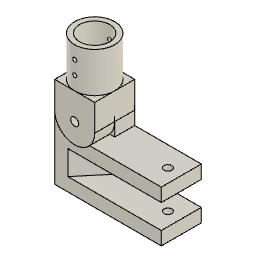
platform-bracket (Autodesk Fusion 360 design; units mm, degrees)
Autodesk Fusion 360 part; units mm, degrees
note: some values were not read from the file. Set by a fixed rule: which face or edge a step refers to.
sketch "Skizze2" plane through (0, 0, 0) normal (0, 0, 1) x (1, 0, 0)
  circle A0 centre (0, 0) radius 11.25
  circle A1 centre (0, 0) radius 15
  dimension "d1" = 22.5
  dimension "d2" = 30
  constraint coincident A0.centre A1.centre
  measures "d1" diameter of A0
  measures "d2" diameter of A1
extrude "Extrusion1" add sketch "Skizze2" along normal blind 30 makes body 1
sketch "Skizze3" plane through (0, 0, 0) normal (0, 0, -1) x (1, 0, 0)
  circle A0 centre (0, 0) radius 11.25
  circle A1 centre (0, 0) radius 15
  line L0 (15, -15) -> (-15, -15)
  line L1 (-15, -15) -> (-15, 15)
  line L2 (-15, 15) -> (15, 15)
  line L3 (15, 15) -> (15, -15)
  line L4 (15, -15) -> (-15, 15) construction
  line L5 (-15, -15) -> (15, 15) construction
  dimension "d5" = 30
  dimension "d6" = 30
  constraint perpendicular L0 L1
  constraint parallel L0 L2
  constraint parallel L1 L3
  constraint horizontal L0
  constraint coincident L4 A0.centre
  constraint coincident L5 A0.centre
  constraint coincident A0.centre A1.centre
  measures "d5" distance of L1.end L2.end
  measures "d6" distance of L0.end L1.end
extrude "Extrusion2" add sketch "Skizze3" along normal blind 5 contours A0 | A1 | A1 L0 L3 | A1 L2 L3 | A1 L1 L2 | A1 L0 L1 bodies 1
sketch "Skizze4" plane through (0, -15, 0) normal (0, -1, 0) x (1, 0, 0)
  line L0 (0, 0) -> (-15, 0)
  line L1 (-15, 0) -> (-15, -5)
  line L2 (-15, -5) -> (15, -5)
  line L3 (15, -5) -> (15, 0)
  line L4 (15, 0) -> (0, 0)
  circle A0 centre (0, -20) radius 15
  line L5 (-15, -5) -> (-15, -20)
  line L6 (15, -5) -> (15, -20)
  circle A1 centre (0, -20) radius 3
  dimension "d9" = 30
  dimension "d10" = 6
  constraint coincident L1.end L2.start
  constraint coincident A0 L5.end
  constraint tangent A0 L5
  constraint perpendicular L2 L5
  constraint coincident L2.end L3.start
  constraint coincident A0 L6.end
  constraint tangent A0 L6
  constraint perpendicular L2 L6
  constraint concentric A0 A1
  measures "d9" diameter of A0
  measures "d10" diameter of A1
extrude "Extrusion3" add sketch "Skizze4" against normal blind 15 contours L2 A0 L5 | L2 A0 L6 | A0 bodies 1
extrude "Extrusion4" add sketch "Skizze4" against normal blind 30 contours L2 A0 L5 | L2 A0 L6 bodies 1
sketch "Skizze5" plane through (0, 0, 0) normal (0, 1, 0) x (-1, 0, 0)
  arc A0 (15, -20) -> (-15, -20) centre (0, -20) ccw
  arc A1 (-15, -20) -> (15, -20) centre (0, -20) ccw
  circle A2 centre (0, -20) radius 3
  circle A3 centre (0, -20) radius 3
  circle A4 centre (0, -20) radius 15
  line L0 (15, -35) -> (-15, -35)
  line L1 (-15, -35) -> (-15, -5)
  line L2 (-15, -5) -> (15, -5)
  line L3 (15, -5) -> (15, -35)
  line L4 (15, -35) -> (-15, -5) construction
  line L5 (-15, -35) -> (15, -5) construction
  point P0 (0, -20)
  dimension "d15" = 30
  dimension "d16" = 30
  constraint concentric A0 A3
  constraint concentric A0 A4
  constraint coincident A0.start A4
  constraint perpendicular L0 L1
  constraint parallel L0 L2
  constraint parallel L1 L3
  constraint horizontal L0
  constraint coincident L4 P0
  constraint coincident L5 P0
  constraint coincident P0 A0.centre
  measures "d15" distance of L0.end L1.end
  measures "d16" distance of L1.end L2.end
extrude "Extrusion5" add sketch "Skizze5" along normal blind 15 separate body contours A0 A1 A4 | A1 A4 L0 L3 | A1 A4 L0 L1 makes body 2
extrude "Extrusion6" add sketch "Skizze5" against normal blind 15 contours A1 A4 L0 L3 | A1 A4 L0 L1 bodies 2
extrude "Extrusion7" add 3 faces at (0, 10, -35) (5, -5, -35) (-10, -10, -35) along direction (0, 0, -1) blind 5 on bodies 2 bodies 2
sketch "Skizze13" plane through (0, -15, 0) normal (0, -1, 0) x (1, 0, 0)
  line L0 (15, -40) -> (15, -20)
  arc A0 (-15, -20) -> (15, -20) centre (0, -20) ccw
  line L1 (-15, -20) -> (-15, -40)
  line L2 (-15, -40) -> (15, -40)
  line L3 (15, -30) -> (11.1803, -30)
  constraint midpoint L0 L3.start
  constraint coincident A0 L3.end
  constraint perpendicular L0 L3
extrude "Extrusion14" cut sketch "Skizze13" against normal blind 15 contours L0 A0 L3 bodies 2
sketch "Skizze14" plane through (15, 0, 0) normal (1, 0, 0) x (0, 1, 0)
  line L0 (0, -20) -> (0, -30)
  line L1 (0, -30) -> (-15, -30)
  line L2 (-15, -30) -> (-15, -40)
  line L3 (-15, -40) -> (15, -40)
  line L4 (15, -40) -> (15, -20)
  line L5 (15, -20) -> (0, -20)
  line L6 (0, -30) -> (15, -30)
  constraint coincident L0.end L1.start
  constraint midpoint L4 L6.end
extrude "Extrusion15" add sketch "Skizze14" along normal blind 50 contours L1 L2 L3 L4 L6 bodies 2
sketch "Skizze15" plane through (0, 0, -40) normal (0, 0, -1) x (1, 0, 0)
  line L0 (-15, 15) -> (-15, -15)
  line L1 (-15, -15) -> (65, -15)
  line L2 (65, -15) -> (65, 15)
  line L3 (65, 15) -> (-15, 15)
  line L4 (-15, 15) -> (-5, 15) construction
  circle A0 centre (577.121, 487.9008) radius 750
  dimension "d53" = 10
  dimension "d54" = 1500
  constraint coincident L0.start L3.end
  constraint perpendicular L0 L4
  constraint coincident L4.end A0
  measures "d53" distance of L0.start L4.end
  measures "d54" diameter of A0
extrude "Extrusion16" add sketch "Skizze15" along normal blind 18.2 contours L0 L1 L3 A0 bodies 2
sketch "Skizze16" plane through (0, 0, -58.2) normal (0, 0, -1) x (1, 0, 0)
  line L0 (-5, 15) -> (-15, 15)
  line L1 (-15, 15) -> (-15, -15)
  line L2 (-15, -15) -> (20.7121, -15)
  arc A0 (-5, 15) -> (20.7121, -15) centre (577.121, 487.9008) ccw
  line L3 (-15, 15) -> (65, 15)
  line L4 (65, 15) -> (65, -15)
  line L5 (65, -15) -> (-15, -15)
  line L6 (-15, -15) -> (-15, 15)
  dimension "d57" = 80
  dimension "d58" = 30
  constraint horizontal L3
  constraint vertical L4
  constraint horizontal L5
  constraint vertical L6
  constraint coincident L0.end L1.start
  measures "d57" distance of L0.end L3.end
  measures "d58" distance of L0.end L1.end
extrude "Extrusion17" add sketch "Skizze16" along normal blind 10 bodies 2
sketch "Skizze17" plane through (0, 0, -68.2) normal (0, 0, -1) x (1, 0, 0)
  line L0 (-15, -15) -> (65, -15)
  line L1 (65, -15) -> (65, 15)
  line L2 (65, 15) -> (-15, 15)
  line L3 (-15, 15) -> (-15, -15)
  line L4 (65, 0) -> (55, 0) construction
  circle A0 centre (55, 0) radius 3
  dimension "d61" = 10
  dimension "d62" = 6
  constraint midpoint L1 L4.start
  constraint perpendicular L1 L4
  constraint coincident L4.end A0.centre
  measures "d61" distance of L4.start L4.end
  measures "d62" diameter of A0
extrude "Extrusion18" cut sketch "Skizze17" against normal blind 40 contours A0 bodies 2
sketch "Skizze18" plane through (0, -15, 0) normal (0, -1, 0) x (1, 0, 0)
  circle A0 centre (0, -20) radius 3
  line L0 (15, -20) -> (15, 0)
  line L1 (15, 0) -> (0, 0)
  line L2 (0, 0) -> (-15, 0)
  line L3 (-15, 0) -> (-15, -20)
  arc A1 (-15, -20) -> (15, -20) centre (0, -20) ccw
  line L4 (0, -20) -> (0, 30.1674) construction
  line L5 (0, 30.1674) -> (0, 20.1674) construction
  circle A2 centre (0, 20.1674) radius 1.5
  line L6 (0, 20.1674) -> (0, 10.1674)
  circle A3 centre (0, 10.1674) radius 1.5
  dimension "d65" = 10
  dimension "d66" = 3
  dimension "d67" = 10
  dimension "d68" = 3
  constraint coincident A0.centre A1.centre
  constraint perpendicular L1 L4
  constraint perpendicular L2 L5
  constraint coincident L5.end A2.centre
  constraint vertical L6
  constraint coincident L6.end A3.centre
  measures "d65" distance of L4.end L5.end
  measures "d66" diameter of A2
  measures "d67" distance of L5.end L6.end
  measures "d68" diameter of A3
extrude "Extrusion19" cut sketch "Skizze18" against normal blind 30 contours A2 | A3 bodies 1
